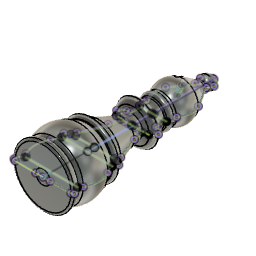
Knight v1 (Autodesk Fusion 360 design; units mm, degrees)
Autodesk Fusion 360 part; units mm, degrees
note: some values were not read from the file. Set by a fixed rule: which sketch regions a step uses.
sketch "SVD" plane through (0, 0, 0) normal (0, 0, 1) x (1, 0, 0)
  line L0 (42.4461, 7.6846) -> (49.4829, 7.6846)
  spline S0 degree 3 poles (49.4829, 7.6846) (49.7483, 7.7788) (49.8565, 7.9987) (49.789, 8.2437) knots 0 0 0 0 1 1 1 1
  spline S1 degree 3 poles (49.789, 8.2437) (49.7202, 8.4932) (49.5062, 8.6292) (49.2093, 8.6265) knots 0 0 0 0 1 1 1 1
  spline S2 degree 3 poles (49.2093, 8.6265) (47.9555, 8.6165) (46.7014, 8.6223) (45.4472, 8.6231) knots 0 0 0 0 1 1 1 1
  spline S3 degree 3 poles (45.4472, 8.6231) (44.5275, 8.6234) (43.6078, 8.6281) (42.6882, 8.626) knots 0 0 0 0 1 1 1 1
  spline S4 degree 3 poles (42.6882, 8.626) (42.345, 8.6249) (42.1675, 8.4217) (42.1669, 8.0995) knots 0 0 0 0 1 1 1 1
  spline S5 degree 3 poles (42.1669, 8.0995) (42.1661, 7.868) (42.2733, 7.7386) (42.4461, 7.6846) knots 0 0 0 0 1 1 1 1
  spline S6 degree 3 poles (48.011, 17.8256) (47.8097, 18.0063) (47.8899, 18.0748) (47.9975, 18.2478) knots 0 0 0 0 1 1 1 1
  spline S7 degree 3 poles (47.9975, 18.2478) (48.5704, 19.1673) (48.7844, 20.1134) (48.2177, 21.1387) knots 0 0 0 0 1 1 1 1
  spline S8 degree 3 poles (48.2177, 21.1387) (47.7271, 22.0261) (47.1752, 22.8698) (46.5693, 23.68) knots 0 0 0 0 1 1 1 1
  spline S9 degree 3 poles (46.5693, 23.68) (46.4799, 23.7991) (46.4315, 23.894) (46.4611, 24.0052) knots 0 0 0 0 1 1 1 1
  spline S10 degree 3 poles (46.4611, 24.0052) (46.6942, 24.1576) (46.8487, 24.4206) (46.8487, 24.7201) knots 0 0 0 0 1 1 1 1
  spline S11 degree 3 poles (46.8487, 24.7201) (46.8487, 25.1918) (46.4667, 25.5741) (45.9947, 25.5741) knots 0 0 0 0 1 1 1 1
  spline S12 degree 3 poles (45.9947, 25.5741) (45.5226, 25.5741) (45.1406, 25.1918) (45.1406, 24.7201) knots 0 0 0 0 1 1 1 1
  spline S13 degree 3 poles (45.1406, 24.7201) (45.1406, 24.4224) (45.2932, 24.1605) (45.524, 24.0078) knots 0 0 0 0 1 1 1 1
  spline S14 degree 3 poles (45.524, 24.0078) (45.5451, 23.8141) (45.4097, 23.658) (45.2816, 23.4808) knots 0 0 0 0 1 1 1 1
  spline S15 degree 3 poles (45.2816, 23.4808) (45.1837, 23.3453) (45.0914, 23.2048) (44.9832, 23.0778) knots 0 0 0 0 1 1 1 1
  spline S16 degree 3 poles (44.9832, 23.0778) (44.7585, 22.8151) (44.7204, 22.5568) (44.8969, 22.2385) knots 0 0 0 0 1 1 1 1
  spline S17 degree 3 poles (44.8969, 22.2385) (45.0914, 21.8864) (45.2379, 21.5067) (45.3983, 21.136) knots 0 0 0 0 1 1 1 1
  spline S18 degree 3 poles (45.3983, 21.136) (45.4335, 21.0548) (45.5031, 20.9384) (45.3697, 20.8849) knots 0 0 0 0 1 1 1 1
  spline S19 degree 3 poles (45.3697, 20.8849) (45.2583, 20.8405) (45.1916, 20.9352) (45.1443, 21.0231) knots 0 0 0 0 1 1 1 1
  spline S20 degree 3 poles (45.1443, 21.0231) (45.1054, 21.0966) (45.0855, 21.1815) (45.0422, 21.2524) knots 0 0 0 0 1 1 1 1
  spline S21 degree 3 poles (45.0422, 21.2524) (44.8429, 21.576) (44.7831, 21.9774) (44.5043, 22.2748) knots 0 0 0 0 1 1 1 1
  spline S22 degree 3 poles (44.5043, 22.2748) (44.3569, 22.0843) (44.2066, 21.9343) (44.1098, 21.7554) knots 0 0 0 0 1 1 1 1
  spline S23 degree 3 poles (44.1098, 21.7554) (43.7999, 21.1821) (43.3594, 20.6741) (43.4147, 19.9367) knots 0 0 0 0 1 1 1 1
  spline S24 degree 3 poles (43.4147, 19.9367) (43.465, 19.2736) (43.6907, 18.7024) (44.051, 18.1671) knots 0 0 0 0 1 1 1 1
  spline S25 degree 3 poles (44.051, 18.1671) (44.1082, 18.0825) (44.1714, 18.0325) (44.0949, 17.9184) knots 0 0 0 0 1 1 1 1
  spline S26 degree 3 poles (44.0949, 17.9184) (43.7608, 17.4205) (43.7682, 17.1919) (44.2555, 17.0363) knots 0 0 0 0 1 1 1 1
  line L1 (44.2555, 17.0363) -> (47.8253, 17.0363)
  spline S27 degree 3 poles (47.8253, 17.0363) (47.8306, 17.0382) (47.8354, 17.0398) (47.8401, 17.0421) knots 0 0 0 0 1 1 1 1
  spline S28 degree 3 poles (47.8401, 17.0421) (48.2052, 17.225) (48.301, 17.5655) (48.011, 17.8256) knots 0 0 0 0 1 1 1 1
  line L2 (42.2132, 2.6485) -> (49.5546, 2.6485)
  spline S29 degree 3 poles (49.5546, 2.6485) (49.739, 2.6877) (49.8623, 2.7954) (49.9653, 3.0041) knots 0 0 0 0 1 1 1 1
  spline S30 degree 3 poles (49.9653, 3.0041) (50.5439, 4.1786) (50.5542, 5.3362) (49.975, 6.5173) knots 0 0 0 0 1 1 1 1
  spline S31 degree 3 poles (49.975, 6.5173) (49.8094, 6.8554) (49.5631, 7.1605) (49.4718, 7.5343) knots 0 0 0 0 1 1 1 1
  line L3 (49.4718, 7.5343) -> (43.2935, 7.5343)
  spline S32 degree 3 poles (43.2935, 7.5343) (43.2663, 7.5314) (43.2401, 7.5314) (43.2139, 7.5343) knots 0 0 0 0 1 1 1 1
  line L4 (43.2139, 7.5343) -> (42.7167, 7.5343)
  spline S33 degree 3 poles (42.7167, 7.5343) (42.3918, 7.4393) (42.209, 7.1345) (42.0055, 6.7781) knots 0 0 0 0 1 1 1 1
  spline S34 degree 3 poles (42.0055, 6.7781) (41.3091, 5.5582) (41.2433, 4.3445) (41.8023, 3.0711) knots 0 0 0 0 1 1 1 1
  spline S35 degree 3 poles (41.8023, 3.0711) (41.8997, 2.8491) (42.0161, 2.6993) (42.2132, 2.6485) knots 0 0 0 0 1 1 1 1
  line L5 (49.6456, 2.4985) -> (44.3741, 2.4985)
  spline S36 degree 3 poles (44.3741, 2.4985) (44.2294, 2.4861) (44.0804, 2.4776) (43.9312, 2.4985) knots 0 0 0 0 1 1 1 1
  line L6 (43.9312, 2.4985) -> (42.2765, 2.4985)
  spline S37 degree 3 poles (42.2765, 2.4985) (41.8447, 2.4379) (41.674, 2.2458) (41.6206, 1.7593) knots 0 0 0 0 1 1 1 1
  spline S38 degree 3 poles (41.6206, 1.7593) (41.5907, 1.483) (41.6558, 1.3642) (41.9772, 1.3669) knots 0 0 0 0 1 1 1 1
  spline S39 degree 3 poles (41.9772, 1.3669) (43.6153, 1.3812) (45.2541, 1.3661) (46.8927, 1.365) knots 0 0 0 0 1 1 1 1
  spline S40 degree 3 poles (46.8927, 1.365) (47.8798, 1.364) (48.8678, 1.3685) (49.8547, 1.3727) knots 0 0 0 0 1 1 1 1
  spline S41 degree 3 poles (49.8547, 1.3727) (49.9856, 1.373) (50.1304, 1.3277) (50.1724, 1.5418) knots 0 0 0 0 1 1 1 1
  spline S42 degree 3 poles (50.1724, 1.5418) (50.2499, 1.9365) (50.0057, 2.3755) (49.6456, 2.4985) knots 0 0 0 0 1 1 1 1
  spline S43 degree 3 poles (48.9982, 9.3049) (48.4987, 10.3323) (48.073, 11.3838) (47.7568, 12.4876) knots 0 0 0 0 1 1 1 1
  spline S44 degree 3 poles (47.7568, 12.4876) (47.6187, 12.9694) (47.6179, 13.4753) (47.4414, 13.9791) knots 0 0 0 0 1 1 1 1
  line L7 (47.4414, 13.9791) -> (46.9191, 13.9791)
  spline S45 degree 3 poles (46.9191, 13.9791) (46.7127, 13.9719) (46.5061, 13.9732) (46.2997, 13.9791) knots 0 0 0 0 1 1 1 1
  line L8 (46.2997, 13.9791) -> (45.3872, 13.9791)
  spline S46 degree 3 poles (45.3872, 13.9791) (45.2374, 13.9574) (45.0842, 13.9706) (44.9323, 13.9791) knots 0 0 0 0 1 1 1 1
  line L9 (44.9323, 13.9791) -> (44.708, 13.9791)
  spline S47 degree 3 poles (44.708, 13.9791) (44.5519, 13.9603) (44.4712, 13.8796) (44.4601, 13.6594) knots 0 0 0 0 1 1 1 1
  spline S48 degree 3 poles (44.4601, 13.6594) (44.4373, 13.2141) (44.3399, 12.7757) (44.2111, 12.3474) knots 0 0 0 0 1 1 1 1
  spline S49 degree 3 poles (44.2111, 12.3474) (43.8753, 11.2284) (43.4475, 10.145) (42.9247, 9.0996) knots 0 0 0 0 1 1 1 1
  spline S50 degree 3 poles (42.9247, 9.0996) (42.8326, 8.9152) (42.754, 8.7292) (43.0562, 8.7197) knots 0 0 0 0 1 1 1 1
  spline S51 degree 3 poles (43.0562, 8.7197) (43.6221, 8.7022) (44.1889, 8.717) (44.7553, 8.7199) knots 0 0 0 0 1 1 1 1
  spline S52 degree 3 poles (44.7553, 8.7199) (46.0441, 8.7273) (47.3329, 8.748) (48.6212, 8.7379) knots 0 0 0 0 1 1 1 1
  spline S53 degree 3 poles (48.6212, 8.7379) (49.2374, 8.7332) (49.2668, 8.7527) (48.9982, 9.3049) knots 0 0 0 0 1 1 1 1
  line L10 (43.8282, 14.1296) -> (43.9161, 14.1296)
  line L11 (43.9161, 14.1296) -> (44.2016, 14.1296)
  line L12 (44.2016, 14.1296) -> (45.5512, 14.1296)
  line L13 (45.5512, 14.1296) -> (47.3837, 14.1296)
  line L14 (47.3837, 14.1296) -> (47.9018, 14.1296)
  line L15 (47.9018, 14.1296) -> (48.155, 14.1296)
  line L16 (48.155, 14.1296) -> (48.1999, 14.1296)
  spline S54 degree 3 poles (48.1999, 14.1296) (48.2063, 14.1304) (48.2119, 14.132) (48.2179, 14.1328) knots 0 0 0 0 1 1 1 1
  spline S55 degree 3 poles (48.2179, 14.1328) (48.5696, 14.1648) (48.8447, 14.4598) (48.8447, 14.8199) knots 0 0 0 0 1 1 1 1
  spline S56 degree 3 poles (48.8447, 14.8199) (48.8447, 15.2009) (48.536, 15.5099) (48.155, 15.5099) knots 0 0 0 0 1 1 1 1
  line L17 (48.155, 15.5099) -> (47.739, 15.5099)
  spline S57 degree 3 poles (47.739, 15.5099) (47.7277, 15.5393) (47.72, 15.5763) (47.7166, 15.6234) knots 0 0 0 0 1 1 1 1
  spline S58 degree 3 poles (47.7166, 15.6234) (47.6856, 16.0444) (47.8036, 16.4677) (47.6848, 16.8866) knots 0 0 0 0 1 1 1 1
  line L18 (47.6848, 16.8866) -> (44.3683, 16.8866)
  spline S59 degree 3 poles (44.3683, 16.8866) (44.2558, 16.8117) (44.2624, 16.6937) (44.2632, 16.5791) knots 0 0 0 0 1 1 1 1
  spline S60 degree 3 poles (44.2632, 16.5791) (44.2645, 16.3569) (44.2674, 16.1343) (44.2674, 15.9121) knots 0 0 0 0 1 1 1 1
  spline S61 degree 3 poles (44.2674, 15.9121) (44.2672, 15.7557) (44.268, 15.6118) (44.1957, 15.5097) knots 0 0 0 0 1 1 1 1
  line L19 (44.1957, 15.5097) -> (43.8288, 15.5097)
  spline S62 degree 3 poles (43.8288, 15.5097) (43.4472, 15.5097) (43.1385, 15.2009) (43.1385, 14.8196) knots 0 0 0 0 1 1 1 1
  spline S63 degree 3 poles (43.1385, 14.8196) (43.1385, 14.4384) (43.4464, 14.1296) (43.8282, 14.1296) knots 0 0 0 0 1 1 1 1
  line L20 (45.8839, 2.6485) -> (45.8839, 7.5343)
  line L21 (45.8839, 2.4985) -> (45.8839, 1.3671)
  line L22 (46.0265, 16.8866) -> (46.0265, 14.1296)
  line L23 (45.9947, 25.5741) -> (46.0404, 17.0363)
  line L24 (45.9645, 7.6846) -> (45.9645, 8.6225)
  line L25 (45.9609, 8.7294) -> (45.9863, 13.9791)
  constraint midpoint L2 L20.start
  constraint coincident L3 L20.end
  constraint perpendicular L3 L20
  constraint coincident L5 L21.start
  constraint coincident S39 L21.end
  constraint perpendicular L5 L21
  constraint midpoint L18 L22.start
  constraint coincident L13 L22.end
  constraint perpendicular L18 L22
  constraint midpoint L1 L23.end
  constraint coincident S52 L25.start
  constraint coincident L8 L25.end
revolve "Revolve1" add sketch "SVD" angle 360 about axis through (45.8839, 2.6485, 0) along (0, 1, 0) contours L0 S0 S1 S2 L24 | S6 S7 S8 S9 S10 S11 L1 S27 S28 L23 | L2 S29 S30 S31 L3 L20 | L5 S39 S40 S41 S42 L21 | S43 S44 L7 S45 L8 S52 S53 L25 | L13 L14 L15 L16 S54 S55 S56 L17 S57 S58 L18 L22 makes body 1 at (48.1372, 7.6846, -0.8808) makes body 2 at (44.364, 18.8653, -1.9059) makes body 3 at (43.1583, 3.7461, -3.4179) makes body 4 at (44.2375, 10.3414, -2.0646) makes body 5 at (44.0648, 15.0606, -2.2811) makes body 6 at (48.8527, 1.3686, 0.2971)
sketch "Nebun modificari" plane through (0, 0, 0) normal (0, 0, 1) x (1, 0, 0)
  line L0 (49.6456, 2.4985) -> (42.1222, 2.4985)
  spline S0 degree 3 poles (42.1222, 2.4985) (42.036, 2.469) (41.957, 2.4217) (41.8173, 2.3013) (41.7572, 2.228) (41.6517, 2.0507) (41.6113, 1.9421) (41.5767, 1.7349) (41.5767, 1.637) (41.5954, 1.5418) knots -0.118446 -0.118446 -0.118446 -0.118446 -0.091041 -0.091041 -0.063036 -0.063036 -0.029099 -0.029099 0 0 0 0
  spline S1 degree 3 poles (41.5954, 1.5418) (41.6035, 1.5006) (41.6153, 1.4695) (41.6399, 1.429) (41.6525, 1.4141) (41.6841, 1.3902) (41.7018, 1.3822) (41.7788, 1.3616) (41.8477, 1.3728) (41.9132, 1.3727) knots -0.041795 -0.041795 -0.041795 -0.041795 -0.032657 -0.032657 -0.026172 -0.026172 -0.019648 -0.019648 0 0 0 0
  spline S2 degree 3 poles (41.9132, 1.3727) (42.4062, 1.3706) (42.9004, 1.3684) (43.8877, 1.3654) (44.3815, 1.3645) (44.8752, 1.365) knots -0.296198 -0.296198 -0.296198 -0.296198 -0.148096 -0.148096 0 0 0 0
  spline S3 degree 3 poles (44.8752, 1.365) (45.0433, 1.3651) (45.2114, 1.3654) (45.5471, 1.3661) (45.7146, 1.3666) (45.8827, 1.3671) (45.8833, 1.3671) (45.8839, 1.3671) knots -0.100694 -0.100694 -0.100694 -0.100694 -0.050258 -0.050258 0 0 0.000179 0.000179 0.000179 0.000179
  spline S4 degree 3 poles (45.8839, 1.3671) (45.8845, 1.3671) (45.8851, 1.3671) (46.0532, 1.3666) (46.2208, 1.3661) (46.5564, 1.3654) (46.7245, 1.3651) (46.8927, 1.365) knots -0.100873 -0.100873 -0.100873 -0.100873 -0.100694 -0.100694 -0.050436 -0.050436 0 0 0 0
  spline S5 degree 3 poles (46.8927, 1.365) (47.3863, 1.3645) (47.8801, 1.3654) (48.8674, 1.3684) (49.3616, 1.3706) (49.8547, 1.3727) knots -0.295817 -0.295817 -0.295817 -0.295817 -0.147912 -0.147912 0 0 0 0
  spline S6 degree 3 poles (49.8547, 1.3727) (49.8954, 1.3728) (49.9375, 1.3685) (50.0027, 1.3692) (50.0271, 1.3714) (50.067, 1.3828) (50.0828, 1.39) (50.1139, 1.4125) (50.1271, 1.4278) (50.1524, 1.4691) (50.1643, 1.5003) (50.1724, 1.5418) knots -0.057727 -0.057727 -0.057727 -0.057727 -0.040786 -0.040786 -0.030068 -0.030068 -0.022004 -0.022004 -0.012677 -0.012677 0 0 0 0
  spline S7 degree 3 poles (50.1724, 1.5418) (50.1924, 1.6434) (50.1911, 1.7482) (50.1525, 1.9512) (50.1154, 2.0495) (50.0118, 2.2282) (49.9445, 2.3096) (49.7991, 2.4286) (49.7255, 2.4712) (49.6456, 2.4985) knots -0.118178 -0.118178 -0.118178 -0.118178 -0.087176 -0.087176 -0.056329 -0.056329 -0.025325 -0.025325 0 0 0 0
  line L1 (49.4718, 7.5343) -> (42.296, 7.5343)
  spline S8 degree 3 poles (42.296, 7.5343) (42.2504, 7.3474) (42.166, 7.1777) (41.9785, 6.847) (41.8757, 6.6866) (41.7928, 6.5173) knots -0.113078 -0.113078 -0.113078 -0.113078 -0.056566 -0.056566 0 0 0 0
  spline S9 degree 3 poles (41.7928, 6.5173) (41.6374, 6.2005) (41.5166, 5.8691) (41.374, 5.1978) (41.3491, 4.8689) (41.4075, 3.9984) (41.5645, 3.4874) (41.8026, 3.0041) knots -0.367355 -0.367355 -0.367355 -0.367355 -0.261542 -0.261542 -0.161605 -0.161605 0 0 0 0
  spline S10 degree 3 poles (41.8026, 3.0041) (41.8306, 2.9473) (41.8636, 2.8909) (41.9374, 2.7978) (41.9763, 2.7596) (42.0802, 2.6882) (42.1441, 2.6632) (42.2132, 2.6485) knots -0.056797 -0.056797 -0.056797 -0.056797 -0.037711 -0.037711 -0.021188 -0.021188 0 0 0 0
  line L2 (42.2132, 2.6485) -> (49.5546, 2.6485)
  spline S11 degree 3 poles (49.5546, 2.6485) (49.5987, 2.6579) (49.6414, 2.6716) (49.7216, 2.7103) (49.7574, 2.734) (49.8571, 2.8206) (49.9137, 2.8995) (49.9653, 3.0041) knots -0.070252 -0.070252 -0.070252 -0.070252 -0.052348 -0.052348 -0.034987 -0.034987 0 0 0 0
  spline S12 degree 3 poles (49.9653, 3.0041) (50.1223, 3.323) (50.2454, 3.6565) (50.3921, 4.333) (50.4187, 4.6651) (50.3627, 5.5333) (50.2097, 6.0388) (49.975, 6.5173) knots -0.367406 -0.367406 -0.367406 -0.367406 -0.260817 -0.260817 -0.15987 -0.15987 0 0 0 0
  spline S13 degree 3 poles (49.975, 6.5173) (49.8837, 6.7038) (49.768, 6.8799) (49.5841, 7.2143) (49.5125, 7.3675) (49.4718, 7.5343) knots -0.11412 -0.11412 -0.11412 -0.11412 -0.051533 -0.051533 0 0 0 0
  line L3 (42.2849, 7.6846) -> (45.8034, 7.6846)
  line L4 (45.8034, 7.6846) -> (45.8034, 8.6225)
  spline S14 degree 3 poles (45.8034, 8.6225) (45.2625, 8.6218) (44.7217, 8.6206) (43.6401, 8.6208) (43.0993, 8.6222) (42.5585, 8.6265) knots -0.324484 -0.324484 -0.324484 -0.324484 -0.162234 -0.162234 0 0 0 0
  spline S15 degree 3 poles (42.5585, 8.6265) (42.4941, 8.6271) (42.4293, 8.6212) (42.3105, 8.5932) (42.2561, 8.5729) (42.1527, 8.5128) (42.1061, 8.473) (42.0261, 8.3707) (41.9969, 8.3095) (41.9788, 8.2437) knots -0.075671 -0.075671 -0.075671 -0.075671 -0.05638 -0.05638 -0.039029 -0.039029 -0.02047 -0.02047 0 0 0 0
  spline S16 degree 3 poles (41.9788, 8.2437) (41.9636, 8.1886) (41.9565, 8.1317) (41.9636, 8.0222) (41.9763, 7.9713) (42.0229, 7.8734) (42.0566, 7.8294) (42.152, 7.7439) (42.2165, 7.7089) (42.2849, 7.6846) knots -0.071624 -0.071624 -0.071624 -0.071624 -0.054462 -0.054462 -0.038572 -0.038572 -0.021787 -0.021787 0 0 0 0
  line L5 (45.9645, 7.6846) -> (49.4829, 7.6846)
  spline S17 degree 3 poles (49.4829, 7.6846) (49.543, 7.7059) (49.6002, 7.7355) (49.6922, 7.8093) (49.728, 7.8498) (49.7819, 7.9441) (49.7985, 7.9954) (49.8133, 8.1145) (49.8065, 8.1803) (49.789, 8.2437) knots -0.071529 -0.071529 -0.071529 -0.071529 -0.052403 -0.052403 -0.036083 -0.036083 -0.019735 -0.019735 0 0 0 0
  spline S18 degree 3 poles (49.789, 8.2437) (49.7768, 8.288) (49.7595, 8.3305) (49.7144, 8.408) (49.6877, 8.4423) (49.6076, 8.5197) (49.5501, 8.555) (49.4063, 8.6115) (49.313, 8.6275) (49.2093, 8.6265) knots -0.087541 -0.087541 -0.087541 -0.087541 -0.071055 -0.071055 -0.055392 -0.055392 -0.03109 -0.03109 0 0 0 0
  spline S19 degree 3 poles (49.2093, 8.6265) (48.6686, 8.6222) (48.1278, 8.6208) (47.0462, 8.6206) (46.5053, 8.6218) (45.9645, 8.6225) knots -0.3245 -0.3245 -0.3245 -0.3245 -0.162258 -0.162258 0 0 0 0
  line L6 (45.9645, 8.6225) -> (45.9645, 7.6846)
  spline S20 degree 3 poles (43.1467, 8.7379) (43.59, 8.7414) (44.0334, 8.7412) (44.9201, 8.7372) (45.364, 8.7333) (45.807, 8.7294) knots -0.265794 -0.265794 -0.265794 -0.265794 -0.13291 -0.13291 0 0 0 0
  line L7 (45.807, 8.7294) -> (45.7815, 13.9791)
  line L8 (45.7815, 13.9791) -> (45.4681, 13.9791)
  spline S21 degree 3 poles (45.4681, 13.9791) (45.3649, 13.9761) (45.2617, 13.9744) (45.0552, 13.974) (44.9519, 13.9755) (44.8487, 13.9791) knots -0.061948 -0.061948 -0.061948 -0.061948 -0.030975 -0.030975 0 0 0 0
  line L9 (44.8487, 13.9791) -> (44.3265, 13.9791)
  spline S22 degree 3 poles (44.3265, 13.9791) (44.2381, 13.7268) (44.1938, 13.4742) (44.1149, 12.9754) (44.0801, 12.7285) (44.0111, 12.4876) knots -0.150197 -0.150197 -0.150197 -0.150197 -0.075181 -0.075181 0 0 0 0
  spline S23 degree 3 poles (44.0111, 12.4876) (43.8537, 11.9381) (43.6685, 11.3995) (43.2503, 10.3373) (43.0188, 9.8175) (42.7696, 9.3049) knots -0.342444 -0.342444 -0.342444 -0.342444 -0.170971 -0.170971 0 0 0 0
  spline S24 degree 3 poles (42.7696, 9.3049) (42.6992, 9.1601) (42.6491, 9.0517) (42.6147, 8.9367) (42.6091, 8.9077) (42.6081, 8.8679) (42.6094, 8.8529) (42.6174, 8.8269) (42.623, 8.8162) (42.6402, 8.7952) (42.652, 8.7863) (42.6943, 8.7632) (42.7355, 8.7531) (42.8753, 8.7371) (42.9927, 8.7367) (43.1467, 8.7379) knots -0.187388 -0.187388 -0.187388 -0.187388 -0.134752 -0.134752 -0.11267 -0.11267 -0.099608 -0.099608 -0.088706 -0.088706 -0.075702 -0.075702 -0.046187 -0.046187 0 0 0 0
  spline S25 degree 3 poles (45.9609, 8.7294) (46.4039, 8.7333) (46.8477, 8.7372) (47.7345, 8.7412) (48.1778, 8.7414) (48.6212, 8.7379) knots -0.266031 -0.266031 -0.266031 -0.266031 -0.133002 -0.133002 0 0 0 0
  spline S26 degree 3 poles (48.6212, 8.7379) (48.7953, 8.7366) (48.9227, 8.7372) (49.0429, 8.7566) (49.0702, 8.7639) (49.1052, 8.7798) (49.1178, 8.7874) (49.1374, 8.8059) (49.1445, 8.8157) (49.1559, 8.8408) (49.1586, 8.8556) (49.1606, 8.9009) (49.1536, 8.9377) (49.1138, 9.0623) (49.0652, 9.1671) (48.9982, 9.3049) knots -0.18258 -0.18258 -0.18258 -0.18258 -0.128548 -0.128548 -0.107948 -0.107948 -0.095523 -0.095523 -0.084875 -0.084875 -0.071964 -0.071964 -0.045978 -0.045978 0 0 0 0
  spline S27 degree 3 poles (48.9982, 9.3049) (48.749, 9.8175) (48.5175, 10.3373) (48.0993, 11.3995) (47.9142, 11.9381) (47.7568, 12.4876) knots -0.342436 -0.342436 -0.342436 -0.342436 -0.17147 -0.17147 0 0 0 0
  spline S28 degree 3 poles (47.7568, 12.4876) (47.6877, 12.7285) (47.653, 12.9754) (47.574, 13.4742) (47.5298, 13.7268) (47.4414, 13.9791) knots -0.160537 -0.160537 -0.160537 -0.160537 -0.08018 -0.08018 0 0 0 0
  line L10 (47.4414, 13.9791) -> (46.9191, 13.9791)
  spline S29 degree 3 poles (46.9191, 13.9791) (46.8159, 13.9755) (46.7127, 13.974) (46.5062, 13.9744) (46.4029, 13.9761) (46.2997, 13.9791) knots -0.061948 -0.061948 -0.061948 -0.061948 -0.030973 -0.030973 0 0 0 0
  line L11 (46.2997, 13.9791) -> (45.9863, 13.9791)
  line L12 (45.9863, 13.9791) -> (45.9609, 8.7294)
  line L13 (47.6848, 16.8866) -> (46.0265, 16.8866)
  line L14 (46.0265, 16.8866) -> (46.0265, 14.1296)
  line L15 (46.0265, 14.1296) -> (48.1999, 14.1296)
  spline S30 degree 3 poles (48.1999, 14.1296) (48.2031, 14.13) (48.2061, 14.1306) (48.212, 14.1318) (48.2149, 14.1324) (48.2179, 14.1328) knots -0.001838 -0.001838 -0.001838 -0.001838 -0.00092 -0.00092 0 0 0 0
  spline S31 degree 3 poles (48.2179, 14.1328) (48.301, 14.1403) (48.3815, 14.1627) (48.5292, 14.2346) (48.5952, 14.2826) (48.7126, 14.4042) (48.7613, 14.4788) (48.8279, 14.6431) (48.8447, 14.7307) (48.8447, 14.8199) knots -0.102636 -0.102636 -0.102636 -0.102636 -0.0776 -0.0776 -0.053267 -0.053267 -0.026751 -0.026751 0 0 0 0
  spline S32 degree 3 poles (48.8447, 14.8199) (48.8447, 14.8679) (48.8398, 14.9157) (48.8204, 15.0083) (48.8062, 15.0527) (48.7513, 15.1786) (48.6988, 15.2539) (48.57, 15.378) (48.4954, 15.4267) (48.3313, 15.4931) (48.2439, 15.5099) (48.155, 15.5099) knots -0.108907 -0.108907 -0.108907 -0.108907 -0.094476 -0.094476 -0.080481 -0.080481 -0.053193 -0.053193 -0.026677 -0.026677 0 0 0 0
  line L16 (48.155, 15.5099) -> (47.739, 15.5099)
  spline S33 degree 3 poles (47.739, 15.5099) (47.7328, 15.5261) (47.7282, 15.5431) (47.7207, 15.5808) (47.7181, 15.6024) (47.7166, 15.6234) knots -0.011517 -0.011517 -0.011517 -0.011517 -0.006341 -0.006341 0 0 0 0
  spline S34 degree 3 poles (47.7166, 15.6234) (47.6971, 15.8885) (47.7367, 16.1547) (47.7403, 16.5797) (47.7282, 16.7337) (47.6848, 16.8866) knots -0.126869 -0.126869 -0.126869 -0.126869 -0.047666 -0.047666 0 0 0 0
  line L17 (45.7413, 16.8866) -> (44.083, 16.8866)
  spline S35 degree 3 poles (44.083, 16.8866) (44.0236, 16.6771) (44.0235, 16.4665) (44.045, 16.045) (44.0668, 15.8339) (44.0513, 15.6234) knots -0.126596 -0.126596 -0.126596 -0.126596 -0.063316 -0.063316 0 0 0 0
  spline S36 degree 3 poles (44.0513, 15.6234) (44.0498, 15.6024) (44.0472, 15.5808) (44.0396, 15.5431) (44.0351, 15.5261) (44.0288, 15.5099) knots -0.011552 -0.011552 -0.011552 -0.011552 -0.005192 -0.005192 0 0 0 0
  line L18 (44.0288, 15.5099) -> (43.6129, 15.5099)
  spline S37 degree 3 poles (43.6129, 15.5099) (43.5649, 15.5099) (43.5172, 15.505) (43.4248, 15.4856) (43.3805, 15.4714) (43.2546, 15.4166) (43.1793, 15.3642) (43.0551, 15.2353) (43.0064, 15.1606) (42.94, 14.9964) (42.9231, 14.9089) (42.9231, 14.8199) knots -0.108906 -0.108906 -0.108906 -0.108906 -0.0945 -0.0945 -0.08053 -0.08053 -0.053242 -0.053242 -0.026702 -0.026702 0 0 0 0
  spline S38 degree 3 poles (42.9231, 14.8199) (42.9231, 14.736) (42.938, 14.6534) (42.9963, 14.4997) (43.038, 14.43) (43.1488, 14.3018) (43.2194, 14.2462) (43.3769, 14.1654) (43.462, 14.1408) (43.5499, 14.1328) knots -0.102578 -0.102578 -0.102578 -0.102578 -0.077419 -0.077419 -0.053197 -0.053197 -0.026486 -0.026486 0 0 0 0
  spline S39 degree 3 poles (43.5499, 14.1328) (43.5529, 14.1324) (43.5559, 14.1318) (43.5617, 14.1306) (43.5647, 14.13) (43.5679, 14.1296) knots -0.001924 -0.001924 -0.001924 -0.001924 -0.000961 -0.000961 0 0 0 0
  line L19 (43.5679, 14.1296) -> (45.7413, 14.1296)
  line L20 (45.7413, 14.1296) -> (45.7413, 16.8866)
  spline S40 degree 3 poles (45.7732, 25.5741) (45.7138, 25.5741) (45.6547, 25.5681) (45.5402, 25.544) (45.4852, 25.5265) (45.3295, 25.4587) (45.2363, 25.3938) (45.0826, 25.2345) (45.0223, 25.142) (44.94, 24.9388) (44.9191, 24.8303) (44.9191, 24.7201) knots -0.134836 -0.134836 -0.134836 -0.134836 -0.116986 -0.116986 -0.099681 -0.099681 -0.065921 -0.065921 -0.033079 -0.033079 0 0 0 0
  spline S41 degree 3 poles (44.9191, 24.7201) (44.9191, 24.6325) (44.9323, 24.5458) (44.9843, 24.3819) (45.0217, 24.3058) (45.1329, 24.1447) (45.2135, 24.0661) (45.3067, 24.0052) knots -0.084961 -0.084961 -0.084961 -0.084961 -0.058713 -0.058713 -0.033406 -0.033406 0 0 0 0
  spline S42 degree 3 poles (45.3067, 24.0052) (45.3138, 23.9786) (45.3167, 23.9517) (45.3131, 23.8971) (45.3068, 23.871) (45.2777, 23.7929) (45.2432, 23.7394) (45.1985, 23.68) knots -0.044016 -0.044016 -0.044016 -0.044016 -0.033078 -0.033078 -0.022301 -0.022301 0 0 0 0
  spline S43 degree 3 poles (45.1985, 23.68) (44.8959, 23.2754) (44.6064, 22.8619) (44.0554, 22.0142) (43.7949, 21.5814) (43.5502, 21.1387) knots -0.303322 -0.303322 -0.303322 -0.303322 -0.151753 -0.151753 0 0 0 0
  spline S44 degree 3 poles (43.5502, 21.1387) (43.4053, 20.8767) (43.2997, 20.5984) (43.2044, 20.0338) (43.2079, 19.7658) (43.3318, 19.0685) (43.5176, 18.6534) (43.7703, 18.2478) knots -0.331964 -0.331964 -0.331964 -0.331964 -0.233263 -0.233263 -0.143354 -0.143354 0 0 0 0
  spline S45 degree 3 poles (43.7703, 18.2478) (43.7997, 18.2005) (43.8271, 18.1611) (43.8603, 18.1015) (43.8705, 18.0792) (43.8804, 18.0395) (43.8819, 18.0223) (43.8775, 17.9852) (43.871, 17.965) (43.8399, 17.9089) (43.8072, 17.8708) (43.7568, 17.8256) knots -0.082486 -0.082486 -0.082486 -0.082486 -0.059434 -0.059434 -0.044495 -0.044495 -0.032981 -0.032981 -0.020302 -0.020302 0 0 0 0
  spline S46 degree 3 poles (43.7568, 17.8256) (43.6962, 17.7712) (43.6525, 17.7134) (43.6034, 17.6095) (43.5904, 17.5623) (43.5841, 17.4636) (43.5912, 17.4147) (43.6275, 17.3095) (43.6605, 17.2568) (43.7577, 17.1466) (43.8337, 17.0892) (43.9277, 17.0421) knots -0.115352 -0.115352 -0.115352 -0.115352 -0.091048 -0.091048 -0.072789 -0.072789 -0.054357 -0.054357 -0.031532 -0.031532 0 0 0 0
  spline S47 degree 3 poles (43.9277, 17.0421) (43.9301, 17.041) (43.9325, 17.04) (43.9374, 17.0381) (43.9398, 17.0373) (43.9425, 17.0363) knots -0.001731 -0.001731 -0.001731 -0.001731 -0.000868 -0.000868 0 0 0 0
  line L21 (43.9425, 17.0363) -> (45.7274, 17.0363)
  line L22 (45.7274, 17.0363) -> (45.7732, 25.5741)
  spline S48 degree 3 poles (46.8487, 24.7201) (46.8487, 24.7795) (46.8427, 24.8386) (46.8186, 24.9531) (46.8011, 25.0081) (46.7333, 25.1638) (46.6684, 25.257) (46.5091, 25.4107) (46.4166, 25.4709) (46.2134, 25.5533) (46.1049, 25.5741) (45.9947, 25.5741) knots -0.134838 -0.134838 -0.134838 -0.134838 -0.116986 -0.116986 -0.099676 -0.099676 -0.06592 -0.06592 -0.033087 -0.033087 0 0 0 0
  line L23 (45.9947, 25.5741) -> (46.0404, 17.0363)
  line L24 (46.0404, 17.0363) -> (47.8253, 17.0363)
  spline S49 degree 3 poles (47.8253, 17.0363) (47.828, 17.0373) (47.8304, 17.0381) (47.8354, 17.04) (47.8378, 17.041) (47.8401, 17.0421) knots -0.001591 -0.001591 -0.001591 -0.001591 -0.000793 -0.000793 0 0 0 0
  spline S50 degree 3 poles (47.8401, 17.0421) (47.8888, 17.0665) (47.9356, 17.0951) (48.0168, 17.1582) (48.0523, 17.1919) (48.1168, 17.2722) (48.1444, 17.3197) (48.1768, 17.4165) (48.1834, 17.4633) (48.1778, 17.5624) (48.1639, 17.612) (48.1132, 17.7163) (48.0702, 17.7725) (48.011, 17.8256) knots -0.119119 -0.119119 -0.119119 -0.119119 -0.098983 -0.098983 -0.08101 -0.08101 -0.060756 -0.060756 -0.043061 -0.043061 -0.023832 -0.023832 0 0 0 0
  spline S51 degree 3 poles (48.011, 17.8256) (47.9699, 17.8624) (47.934, 17.9004) (47.9, 17.9583) (47.8929, 17.977) (47.8859, 18.0137) (47.8864, 18.0321) (47.9025, 18.1084) (47.9469, 18.1665) (47.9975, 18.2478) knots -0.064008 -0.064008 -0.064008 -0.064008 -0.047023 -0.047023 -0.038073 -0.038073 -0.028737 -0.028737 0 0 0 0
  spline S52 degree 3 poles (47.9975, 18.2478) (48.2005, 18.5736) (48.3736, 18.9271) (48.5432, 19.5878) (48.5689, 19.8785) (48.498, 20.5164) (48.3842, 20.8374) (48.2177, 21.1387) knots -0.307648 -0.307648 -0.307648 -0.307648 -0.192299 -0.192299 -0.103278 -0.103278 0 0 0 0
  spline S53 degree 3 poles (48.2177, 21.1387) (47.973, 21.5814) (47.7124, 22.0142) (47.1614, 22.8619) (46.8719, 23.2754) (46.5693, 23.68) knots -0.303323 -0.303323 -0.303323 -0.303323 -0.15157 -0.15157 0 0 0 0
  spline S54 degree 3 poles (46.5693, 23.68) (46.5356, 23.7249) (46.5067, 23.7676) (46.4701, 23.8424) (46.4592, 23.8745) (46.4501, 23.9405) (46.4525, 23.9728) (46.4611, 24.0052) knots -0.032665 -0.032665 -0.032665 -0.032665 -0.01994 -0.01994 -0.010049 -0.010049 0 0 0 0
  spline S55 degree 3 poles (46.4611, 24.0052) (46.5336, 24.0525) (46.5985, 24.1107) (46.7091, 24.2446) (46.7541, 24.3198) (46.8279, 24.5022) (46.8487, 24.6102) (46.8487, 24.7201) knots -0.085176 -0.085176 -0.085176 -0.085176 -0.059149 -0.059149 -0.032963 -0.032963 0 0 0 0
  line L25 (42.2132, 2.6485) -> (42.1222, 2.4985)
  line L26 (49.6456, 2.4985) -> (49.5546, 2.6485)
  line L27 (45.8839, 2.4985) -> (45.8839, 2.6485)
  line L28 (42.2849, 7.6846) -> (42.296, 7.5343)
  line L29 (45.8034, 7.6846) -> (45.9645, 7.6846)
  line L30 (45.8839, 7.6846) -> (45.8839, 7.5343)
  line L31 (49.4829, 7.6846) -> (49.4718, 7.5343)
  line L32 (45.8034, 8.6225) -> (45.9645, 8.6225)
  line L33 (45.807, 8.7294) -> (45.9609, 8.7294)
  line L34 (45.8839, 8.7294) -> (45.8839, 8.6225)
  line L35 (43.1467, 8.7379) -> (42.5585, 8.6265)
  line L36 (48.6212, 8.7379) -> (49.2093, 8.6265)
  line L37 (45.7815, 13.9791) -> (45.9863, 13.9791)
  line L38 (45.7413, 14.1296) -> (46.0265, 14.1296)
  line L39 (45.8839, 14.1296) -> (45.8839, 13.9791)
  line L40 (44.3265, 13.9791) -> (43.5679, 14.1296)
  line L41 (47.4414, 13.9791) -> (48.1999, 14.1296)
  line L42 (45.7413, 16.8866) -> (46.0265, 16.8866)
  line L43 (45.7274, 17.0363) -> (46.0404, 17.0363)
  line L44 (45.8839, 17.0363) -> (45.8839, 16.8866)
  line L45 (44.083, 16.8866) -> (43.9425, 17.0363)
  line L46 (47.6848, 16.8866) -> (47.8401, 17.0421)
  spline S56 degree 5 poles (44.3582, 22.48) (44.336, 22.476) (44.3013, 22.4578) (44.2788, 22.3995) (44.308, 22.2595) (44.44, 21.9864) (44.657, 21.6316) (44.9326, 21.236) (45.2279, 20.8576) (45.4651, 20.6154) (45.5782, 20.6011) (45.5738, 20.7798) (45.4807, 21.0813) (45.3364, 21.4275) (45.166, 21.7719) (44.9889, 22.0851) (44.8176, 22.3538) (44.6603, 22.5751) (44.5216, 22.7523) (44.4038, 22.8911) (44.308, 22.995) (44.2493, 23.0519) (44.2153, 23.0803) (44.197, 23.093) (44.189, 23.0977) knots 0 0 0 0 0 0 0.05 0.1 0.15 0.2 0.25 0.3 0.35 0.4 0.45 0.5 0.55 0.6 0.65 0.7 0.75 0.8 0.85 0.9 0.95 1 1 1 1 1 1
  line L47 (44.8642, 21.2888) -> (45.603, 20.448)
  point P0 (45.2336, 20.8684)
  point P1 (45.5, 21)
  point P2 (44.5299, 22.7389)
  constraint coincident S10.end L2.start
  constraint coincident L0.end S0.start
  constraint coincident L0.start S7.end
  constraint coincident L2.end S11.start
  constraint midpoint L0 L27.start
  constraint midpoint L2 L27.end
  constraint coincident L3.start S16.end
  constraint coincident L1.end S8.start
  constraint coincident L3.end L4.start
  constraint coincident L5.start L6.end
  constraint midpoint L29 L30.start
  constraint midpoint L1 L30.end
  constraint coincident L5.end S17.start
  constraint coincident L1.start S13.end
  constraint coincident L4.end S14.start
  constraint coincident S19.end L6.start
  constraint coincident S20.end L7.start
  constraint coincident S25.start L12.end
  constraint midpoint L33 L34.start
  constraint perpendicular L33 L34
  constraint coincident S20.start S24.end
  constraint coincident S14.end S15.start
  constraint coincident S25.end S26.start
  constraint coincident S18.end S19.start
  constraint coincident L7.end L8.start
  constraint coincident L11.end L12.start
  constraint coincident L19.end L20.start
  constraint coincident L14.end L15.start
  constraint midpoint L38 L39.start
  constraint midpoint L37 L39.end
  constraint coincident L9.end S22.start
  constraint coincident S39.end L19.start
  constraint coincident S28.end L10.start
  constraint coincident L15.end S30.start
  constraint coincident L17.start L20.end
  constraint coincident L13.end L14.start
  constraint coincident L21.end L22.start
  constraint coincident L23.end L24.start
  constraint midpoint L43 L44.start
  constraint midpoint L42 L44.end
  constraint coincident L17.end S35.start
  constraint coincident S47.end L21.start
  constraint coincident L13.start S34.end
  constraint coincident S49.end S50.start
  constraint coincident S43 S56.start
  constraint coincident S43 P2
  constraint midpoint P0 L47
revolve "Revolve2" add sketch "Nebun modificari" angle 360 about axis through (45.8839, 2.4985, 0) along (0, 1, 0) contours L0 L2 L26 L27 | L1 L5 L29 L30 L31 | S19 S25 L32 L33 L34 L36 | L10 S29 L11 L15 L37 L38 L39 L41 | L13 L24 S49 L42 L43 L44 L46 bodies 1 2 3 4 5 6
extrude "Extrude1" cut sketch "Nebun modificari" along normal mid plane 7 contours S43 S56 picked at (44.7183, 21.8792) bodies 1
fillet "Fillet1" radius 0.1 6 edges at (45.4871, 20.6405, -2.5204) (44.9098, 22.2052, -1.396) (44.9059, 22.2115, 1.3884) (45.4871, 20.6405, 2.5204) (44.425, 22.0331, 1.0713) (44.4654, 21.9585, -1.1968) on bodies 1
named bodies: "Nebun"
